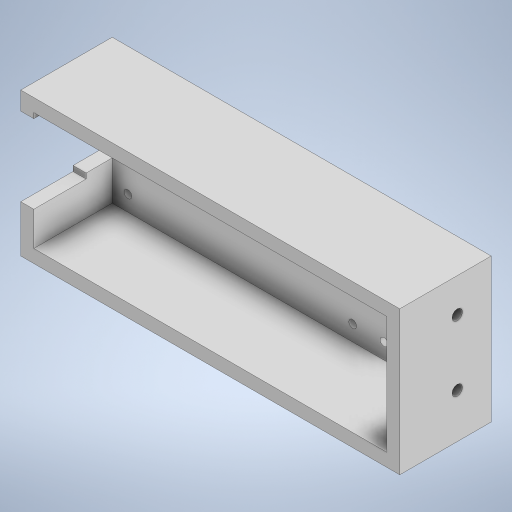
# Autodesk Inventor part: arduino mould_thicker
Saved by Autodesk Inventor 2023 (Build 270158000, 158)
## iProperties
Created: 2023-05-03
Part Number: arduino mould_thicker
Material: Generic
Document SubType Name: Modeling
Designer: gmami
Density: 1 g/cm^3
Appearance: Default
Author: gmami
Autodesk Inventor part; units mm, degrees
ref_plane "YZ Plane" through (0, 0, 0) normal (1, 0, 0) x (0, 1, 0)
ref_plane "XZ Plane" through (0, 0, 0) normal (0, 1, 0) x (-1, 0, 0)
ref_plane "XY Plane" through (0, 0, 0) normal (0, 0, 1) x (1, 0, 0)
sketch "Sketch1" plane through (0, 0, 0) normal (0, 0, 1) x (1, 0, 0)
  line L0 (18.8411, 66.8659) -> (163.8411, 66.8659)
  line L1 (163.8411, 66.8659) -> (163.8411, 11.8659)
  line L2 (163.8411, 11.8659) -> (18.8411, 11.8659)
  line L3 (18.8411, 11.8659) -> (18.8411, 66.8659)
  point P0 (0, 0)
  dimension "d0" = 55
  dimension "d1" = 145
  constraints: 8 end point, 2 parallel, 1 horizontal, 1 perpendicular
  measures "d0" distance of L2.end L0.start
  measures "d1" distance of L0.start L0.end
extrude "Extrusion1" add sketch "Sketch1" along normal blind 35
sketch "Sketch2" plane through (0, 0, 35) normal (0, 0, 1) x (1, 0, 0)
  line L0 (23.8411, 61.8659) -> (158.8411, 61.8659)
  line L1 (158.8411, 61.8659) -> (158.8411, 16.8659)
  line L2 (158.8411, 16.8659) -> (23.8411, 16.8659)
  line L3 (23.8411, 16.8659) -> (23.8411, 61.8659)
  line L4 (18.8411, 66.8659) -> (18.8411, 11.8659) projected
  line L5 (163.8411, 66.8659) -> (18.8411, 66.8659) projected
  line L6 (163.8411, 11.8659) -> (163.8411, 66.8659) projected
  line L7 (18.8411, 11.8659) -> (163.8411, 11.8659) projected
  point P0 (0, 0)
  dimension "d4" = 5
  dimension "d5" = 5
  dimension "d6" = 5
  dimension "d7" = 5
  constraints: 8 end point, 2 parallel, 1 horizontal, 1 perpendicular
  measures "d4" distance between parallel lines of L4 L3
  measures "d5" distance between parallel lines of L5 L0
  measures "d6" distance between parallel lines of L6 L1
  measures "d7" distance between parallel lines of L2 L7
extrude "Extrusion2" cut sketch "Sketch2" against normal blind 30 contours L0 L1 L2 L3
sketch "Sketch3" plane through (0, 0, 0) normal (0, 0, -1) x (-1, 0, 0)
  circle A0 centre (-29.8411, 22.8659) radius 1.5
  circle A1 centre (-29.8411, 55.8659) radius 1.5
  line L0 (-18.8411, 66.8659) -> (-18.8411, 11.8659) projected
  line L1 (-18.8411, 11.8659) -> (-163.8411, 11.8659) projected
  line L2 (-163.8411, 66.8659) -> (-18.8411, 66.8659) projected
  circle A2 centre (-127.8411, 55.8659) radius 1.5
  circle A3 centre (-127.8411, 22.8659) radius 1.5
  line L3 (-163.8411, 11.8659) -> (-163.8411, 66.8659) projected
  circle A4 centre (-115.8411, 55.8659) radius 1.5
  circle A5 centre (-115.8411, 22.8659) radius 1.5
  point P0 (0, 0)
  dimension "d10" = 3
  dimension "d11" = 11
  dimension "d12" = 11
  dimension "d13" = 11
  dimension "d14" = 11
  dimension "d15" = 3
  dimension "d19" = 3
  dimension "d20" = 3
  dimension "d24" = 36
  dimension "d26" = 12
  dimension "d27" = 36
  dimension "d28" = 12
  dimension "d29" = 3
  dimension "d30" = 3
  dimension "d31" = 11
  dimension "d32" = 11
  dimension "d33" = 11
  dimension "d34" = 11
  constraints: 6 centre point
  measures "d10" diameter of A0
  measures "d11" distance from line of L0 A0.centre
  measures "d12" distance from line of A0.centre L1
  measures "d13" distance from line of L0 A1.centre
  measures "d14" distance from line of L2 A1.centre
  measures "d15" diameter of A1
  measures "d19" diameter of A2
  measures "d20" diameter of A3
  measures "d24" distance from line of L3 A2.centre
  measures "d26" distance of A4.centre A2.centre
  measures "d27" distance from line of L3 A3.centre
  measures "d28" distance of A3.centre A5.centre
  measures "d29" diameter of A4
  measures "d30" diameter of A5
  measures "d31" distance from line of L2 A2.centre
  measures "d32" distance from line of L2 A4.centre
  measures "d33" distance from line of L1 A5.centre
  measures "d34" distance from line of L1 A3.centre
extrude "Extrusion3" cut sketch "Sketch3" against normal blind 30 contours A0 | A1 | A2 | A3 | A4 | A5
sketch "Sketch4" plane through (18.8411, 11.8659, 0) normal (-1, 0, 0) x (0, 0, 1)
  line L0 (35, 0) -> (35, 55) projected
  line L1 (35, 48) -> (15, 48)
  line L2 (15, 48) -> (15, 18)
  line L3 (15, 18) -> (35, 18)
  line L4 (35, 18) -> (35, 48)
  line L5 (0, 55) -> (35, 55) projected
  line L6 (15, 20) -> (15, 40)
  line L7 (15, 45) -> (5, 45)
  line L8 (5, 45) -> (5, 20)
  line L9 (5, 20) -> (15, 20)
  line L10 (15, 20) -> (15, 45)
  line L11 (0, 55) -> (0, 0) projected
  point P0 (0, -11.8659)
  point P1 (35, 18)
  point P2 (15, 20)
  point P3 (15, 20)
  dimension "d37" = 7
  dimension "d38" = 30
  dimension "d44" = 10
  dimension "d45" = 25
  dimension "d46" = 5
  dimension "d47" = 15
  constraints: 18 end point, 4 parallel, 2 horizontal, 2 perpendicular, 2 point on line
  measures "d37" distance between parallel lines of L5 L1
  measures "d38" distance between parallel lines of L1 L3
  measures "d44" distance between parallel lines of L5 L7
  measures "d45" distance between parallel lines of L7 L9
  measures "d46" distance between parallel lines of L11 L8
  measures "d47" distance between parallel lines of L11 L2
extrude "Extrusion4" cut sketch "Sketch4" against normal blind 30
sketch "Sketch5" plane through (163.8411, 11.8659, 0) normal (1, 0, 0) x (0, 0, -1)
  circle A0 centre (-13, 17) radius 2
  circle A1 centre (-13, 42) radius 2
  line L0 (0, 0) -> (0, 55) projected
  line L1 (0, 0) -> (-35, 0) projected
  dimension "d48" = 4
  dimension "d49" = 4
  dimension "d50" = 25
  dimension "d51" = 13
  dimension "d52" = 13
  dimension "d53" = 17
  constraints: 2 centre point
  measures "d48" diameter of A0
  measures "d49" diameter of A1
  measures "d50" distance of A1.centre A0.centre
  measures "d51" distance from line of L0 A1.centre
  measures "d52" distance from line of L0 A0.centre
  measures "d53" distance from line of L1 A0.centre
extrude "Extrusion5" cut sketch "Sketch5" against normal blind 30
body "Solid1"
